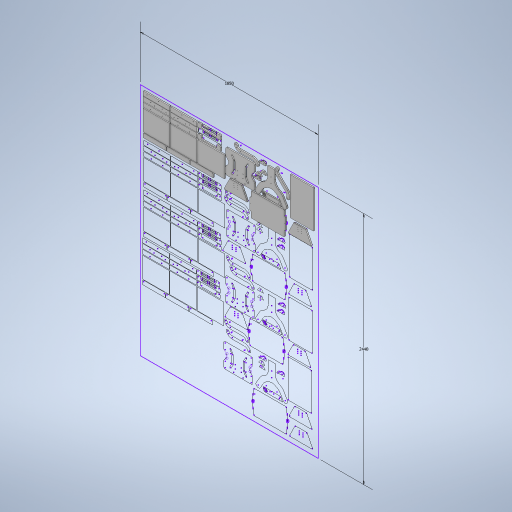
# Autodesk Inventor part: Generador_de_Piezas
Saved by Autodesk Inventor 2024 (Build 280153000, 153)
## iProperties
Created: 2023-05-11
Part Number: Generador_de_Piezas
Material: Genérico
Document SubType Name: Modeling
Designer: sebas
Density: 1 g/cm^3
Appearance: Valor por defecto
Autodesk Inventor part; units mm, degrees
(part 1 of 3)
ref_plane "YZ Plane" through (0, 0, 0) normal (1, 0, 0) x (0, 1, 0)
ref_plane "XZ Plane" through (0, 0, 0) normal (0, 1, 0) x (-1, 0, 0)
ref_plane "XY Plane" through (0, 0, 0) normal (0, 0, 1) x (1, 0, 0)
sketch "Visible" plane through (0, 0, 0) normal (0, 0, 1) x (1, 0, 0)
  line L0 (806.8508, 2400.0345) -> (806.8508, 2412.0345)
  line L1 (646.8508, 2412.0345) -> (619.3508, 2412.0345)
  arc A0 (619.3508, 2412.0345) -> (607.3508, 2400.0345) centre (619.3508, 2400.0345) ccw
  line L2 (646.8508, 2400.0345) -> (646.8508, 2412.0345)
  line L3 (318.2665, 2316.0113) -> (318.2665, 2349.0113)
  line L4 (43.2665, 2316.0113) -> (318.2665, 2316.0113)
  line L5 (43.2665, 2316.0113) -> (43.2665, 2349.0113)
  circle A1 centre (280.5665, 2332.5113) radius 3
  circle A2 centre (160.9665, 2332.5113) radius 3
  circle A3 centre (240.5665, 2343.5113) radius 3
  circle A4 centre (120.9665, 2343.5113) radius 3
  line L6 (318.2665, 2361.0113) -> (318.2665, 2349.0113)
  line L7 (43.2665, 2361.0113) -> (43.2665, 2349.0113)
  line L8 (43.2665, 2361.0113) -> (318.2665, 2361.0113)
  line L9 (600.4289, 2410.0964) -> (600.4289, 2398.0964)
  line L10 (325.4289, 2410.0964) -> (325.4289, 2398.0964)
  line L11 (325.4289, 2410.0964) -> (600.4289, 2410.0964)
  line L12 (600.4289, 2365.0964) -> (600.4289, 2398.0964)
  line L13 (325.4289, 2365.0964) -> (600.4289, 2365.0964)
  line L14 (325.4289, 2365.0964) -> (325.4289, 2398.0964)
  circle A5 centre (562.7289, 2392.5964) radius 3
  circle A6 centre (443.1289, 2392.5964) radius 3
  line L15 (325.2528, 2315.2709) -> (325.2528, 2348.2709)
  line L16 (600.2528, 2315.2709) -> (600.2528, 2348.2709)
  line L17 (600.2528, 2315.2709) -> (325.2528, 2315.2709)
  circle A7 centre (522.5528, 2342.7709) radius 3
  circle A8 centre (402.9528, 2342.7709) radius 3
  circle A9 centre (482.5528, 2331.7709) radius 3
  circle A10 centre (362.9528, 2331.7709) radius 3
  line L18 (325.2528, 2348.2709) -> (325.2528, 2360.2709)
  line L19 (600.2528, 2360.2709) -> (325.2528, 2360.2709)
  line L20 (600.2528, 2348.2709) -> (600.2528, 2360.2709)
  line L21 (799.3625, 2328.4857) -> (659.3625, 2328.4857)
  arc A11 (799.3625, 2328.4857) -> (809.3625, 2338.4857) centre (799.3625, 2338.4857) ccw
  line L22 (809.3625, 2338.4857) -> (809.3625, 2349.4857)
  line L23 (848.8625, 2349.4857) -> (848.8625, 2316.4857)
  line L24 (848.8625, 2316.4857) -> (609.8625, 2316.4857)
  line L25 (609.8625, 2349.4857) -> (609.8625, 2316.4857)
  arc A12 (649.3625, 2338.4857) -> (659.3625, 2328.4857) centre (659.3625, 2338.4857) ccw
  line L26 (649.3625, 2338.4857) -> (649.3625, 2349.4857)
  line L27 (836.8625, 2361.4857) -> (809.3625, 2361.4857)
  arc A13 (848.8625, 2349.4857) -> (836.8625, 2361.4857) centre (836.8625, 2349.4857) ccw
  line L28 (809.3625, 2349.4857) -> (809.3625, 2361.4857)
  line L29 (649.3625, 2361.4857) -> (621.8625, 2361.4857)
  arc A14 (621.8625, 2361.4857) -> (609.8625, 2349.4857) centre (621.8625, 2349.4857) ccw
  line L30 (649.3625, 2349.4857) -> (649.3625, 2361.4857)
  line L31 (42.474, 2263.6267) -> (42.474, 2296.6267)
  line L32 (317.474, 2263.6267) -> (317.474, 2296.6267)
  line L33 (317.474, 2263.6267) -> (42.474, 2263.6267)
  circle A15 centre (239.774, 2280.1267) radius 3
  circle A16 centre (120.174, 2280.1267) radius 3
  line L34 (42.474, 2296.6267) -> (42.474, 2308.6267)
  line L35 (317.474, 2308.6267) -> (42.474, 2308.6267)
  line L36 (317.474, 2296.6267) -> (317.474, 2308.6267)
  line L37 (600.3648, 2308.6267) -> (600.3648, 2296.6267)
  line L38 (325.3648, 2308.6267) -> (325.3648, 2296.6267)
  line L39 (325.3648, 2308.6267) -> (600.3648, 2308.6267)
  line L40 (600.3648, 2263.6267) -> (600.3648, 2296.6267)
  line L41 (325.3648, 2263.6267) -> (600.3648, 2263.6267)
  line L42 (325.3648, 2263.6267) -> (325.3648, 2296.6267)
  circle A17 centre (522.6648, 2280.1267) radius 3
  circle A18 centre (403.0648, 2280.1267) radius 3
  line L43 (797.9907, 2277.247) -> (657.9907, 2277.247)
  arc A19 (797.9907, 2277.247) -> (807.9907, 2287.247) centre (797.9907, 2287.247) ccw
  line L44 (807.9907, 2287.247) -> (807.9907, 2298.247)
  line L45 (847.4907, 2298.247) -> (847.4907, 2265.247)
  line L46 (847.4907, 2265.247) -> (608.4907, 2265.247)
  line L47 (608.4907, 2298.247) -> (608.4907, 2265.247)
  arc A20 (647.9907, 2287.247) -> (657.9907, 2277.247) centre (657.9907, 2287.247) ccw
  line L48 (647.9907, 2287.247) -> (647.9907, 2298.247)
  line L49 (835.4907, 2310.247) -> (807.9907, 2310.247)
  arc A21 (847.4907, 2298.247) -> (835.4907, 2310.247) centre (835.4907, 2298.247) ccw
  line L50 (807.9907, 2298.247) -> (807.9907, 2310.247)
  line L51 (647.9907, 2310.247) -> (620.4907, 2310.247)
  arc A22 (620.4907, 2310.247) -> (608.4907, 2298.247) centre (620.4907, 2298.247) ccw
  line L52 (647.9907, 2298.247) -> (647.9907, 2310.247)
  line L53 (318.3532, 2039.3982) -> (43.3532, 2039.3982)
  line L54 (318.3532, 2039.3982) -> (318.3532, 2254.3982)
  line L55 (43.3532, 2254.3982) -> (43.3532, 2039.3982)
  line L56 (318.3532, 2254.3982) -> (43.3532, 2254.3982)
  line L57 (600.1736, 2040.7797) -> (325.1736, 2040.7797)
  line L58 (600.1736, 2040.7797) -> (600.1736, 2255.7797)
  line L59 (325.1736, 2255.7797) -> (325.1736, 2040.7797)
  line L60 (600.1736, 2255.7797) -> (325.1736, 2255.7797)
  line L61 (885.3014, 2039.5398) -> (610.3014, 2039.5398)
  line L62 (885.3014, 2039.5398) -> (885.3014, 2254.5398)
  line L63 (610.3014, 2254.5398) -> (610.3014, 2039.5398)
  line L64 (885.3014, 2254.5398) -> (610.3014, 2254.5398)
  line L65 (41.6152, 1989.403) -> (280.6152, 1989.403)
  line L66 (41.6152, 2022.403) -> (41.6152, 1989.403)
  line L67 (280.6152, 2022.403) -> (280.6152, 1989.403)
  line L68 (53.6152, 2034.403) -> (268.6152, 2034.403)
  arc A23 (280.6152, 2022.403) -> (268.6152, 2034.403) centre (268.6152, 2022.403) ccw
  arc A24 (53.6152, 2034.403) -> (41.6152, 2022.403) centre (53.6152, 2022.403) ccw
  line L69 (286.1359, 1989.403) -> (525.1359, 1989.403)
  line L70 (286.1359, 2022.403) -> (286.1359, 1989.403)
  line L71 (525.1359, 2022.403) -> (525.1359, 1989.403)
  line L72 (298.1359, 2034.403) -> (513.1359, 2034.403)
  arc A25 (525.1359, 2022.403) -> (513.1359, 2034.403) centre (513.1359, 2022.403) ccw
  arc A26 (298.1359, 2034.403) -> (286.1359, 2022.403) centre (298.1359, 2022.403) ccw
  line L73 (529.3629, 1989.8327) -> (768.3629, 1989.8327)
  line L74 (529.3629, 2022.8327) -> (529.3629, 1989.8327)
  line L75 (768.3629, 2022.8327) -> (768.3629, 1989.8327)
  line L76 (541.3629, 2034.8327) -> (756.3629, 2034.8327)
  arc A27 (768.3629, 2022.8327) -> (756.3629, 2034.8327) centre (756.3629, 2022.8327) ccw
  arc A28 (541.3629, 2034.8327) -> (529.3629, 2022.8327) centre (541.3629, 2022.8327) ccw
  circle A29 centre (717.6352, 2406.9048) radius 3
  circle A30 centre (657.8352, 2406.9048) radius 3
  arc A31 (717.6352, 2401.9048) -> (717.6352, 2411.9048) centre (717.6352, 2406.9048) ccw
  line L77 (717.6352, 2401.9048) -> (657.8352, 2401.9048)
  arc A32 (657.8352, 2411.9048) -> (657.8352, 2401.9048) centre (657.8352, 2406.9048) ccw
  line L78 (717.6352, 2411.9048) -> (657.8352, 2411.9048)
  circle A33 centre (792.7319, 2407.0384) radius 3
  circle A34 centre (732.9319, 2407.0384) radius 3
  arc A35 (792.7319, 2402.0384) -> (792.7319, 2412.0384) centre (792.7319, 2407.0384) ccw
  line L79 (792.7319, 2402.0384) -> (732.9319, 2402.0384)
  arc A36 (732.9319, 2412.0384) -> (732.9319, 2402.0384) centre (732.9319, 2407.0384) ccw
  line L80 (792.7319, 2412.0384) -> (732.9319, 2412.0384)
  circle A37 centre (717.9632, 2391.8594) radius 3
  circle A38 centre (658.1632, 2391.8594) radius 3
  arc A39 (717.9632, 2386.8594) -> (717.9632, 2396.8594) centre (717.9632, 2391.8594) ccw
  line L81 (717.9632, 2386.8594) -> (658.1632, 2386.8594)
  arc A40 (658.1632, 2396.8594) -> (658.1632, 2386.8594) centre (658.1632, 2391.8594) ccw
  line L82 (717.9632, 2396.8594) -> (658.1632, 2396.8594)
  circle A41 centre (793.0598, 2391.993) radius 3
  circle A42 centre (733.2598, 2391.993) radius 3
  arc A43 (793.0598, 2386.993) -> (793.0598, 2396.993) centre (793.0598, 2391.993) ccw
  line L83 (793.0598, 2386.993) -> (733.2598, 2386.993)
  arc A44 (733.2598, 2396.993) -> (733.2598, 2386.993) centre (733.2598, 2391.993) ccw
  line L84 (793.0598, 2396.993) -> (733.2598, 2396.993)
  circle A45 centre (720.4706, 2355.6151) radius 3
  circle A46 centre (660.6706, 2355.6151) radius 3
  arc A47 (720.4706, 2350.6151) -> (720.4706, 2360.6151) centre (720.4706, 2355.6151) ccw
  line L85 (720.4706, 2350.6151) -> (660.6706, 2350.6151)
  arc A48 (660.6706, 2360.6151) -> (660.6706, 2350.6151) centre (660.6706, 2355.6151) ccw
  line L86 (720.4706, 2360.6151) -> (660.6706, 2360.6151)
  circle A49 centre (795.5673, 2355.7486) radius 3
  circle A50 centre (735.7673, 2355.7486) radius 3
  arc A51 (795.5673, 2350.7486) -> (795.5673, 2360.7486) centre (795.5673, 2355.7486) ccw
  line L87 (795.5673, 2350.7486) -> (735.7673, 2350.7486)
  arc A52 (735.7673, 2360.7486) -> (735.7673, 2350.7486) centre (735.7673, 2355.7486) ccw
  line L88 (795.5673, 2360.7486) -> (735.7673, 2360.7486)
  circle A53 centre (720.7986, 2340.5697) radius 3
  circle A54 centre (660.9986, 2340.5697) radius 3
  arc A55 (720.7986, 2335.5697) -> (720.7986, 2345.5697) centre (720.7986, 2340.5697) ccw
  line L89 (720.7986, 2335.5697) -> (660.9986, 2335.5697)
  arc A56 (660.9986, 2345.5697) -> (660.9986, 2335.5697) centre (660.9986, 2340.5697) ccw
  line L90 (720.7986, 2345.5697) -> (660.9986, 2345.5697)
  circle A57 centre (795.8952, 2340.7033) radius 3
  circle A58 centre (736.0952, 2340.7033) radius 3
  arc A59 (795.8952, 2335.7033) -> (795.8952, 2345.7033) centre (795.8952, 2340.7033) ccw
  line L91 (795.8952, 2335.7033) -> (736.0952, 2335.7033)
  arc A60 (736.0952, 2345.7033) -> (736.0952, 2335.7033) centre (736.0952, 2340.7033) ccw
  line L92 (795.8952, 2345.7033) -> (736.0952, 2345.7033)
  circle A61 centre (1238.5575, 2262.083) radius 2.5
  line L93 (1251.0575, 2275.083) -> (1226.0575, 2275.083)
  line L94 (1270.5575, 2247.083) -> (1251.0575, 2275.083)
  line L95 (1206.5575, 2247.083) -> (1270.5575, 2247.083)
  line L96 (1226.0575, 2275.083) -> (1206.5575, 2247.083)
  circle A62 centre (1288.1866, 2298.632) radius 2.5
  line L97 (1300.6866, 2311.632) -> (1275.6866, 2311.632)
  line L98 (1320.1866, 2283.632) -> (1300.6866, 2311.632)
  line L99 (1256.1866, 2283.632) -> (1320.1866, 2283.632)
  line L100 (1275.6866, 2311.632) -> (1256.1866, 2283.632)
  line L101 (1478.5889, 2086.2932) -> (1289.2629, 2086.2932)
  line L102 (1289.2629, 2086.2932) -> (1276.499, 2111.8211)
  arc A63 (1285.4432, 2126.2932) -> (1276.499, 2111.8211) centre (1285.4432, 2116.2932) ccw
  line L103 (1285.4432, 2126.2932) -> (1452.4086, 2126.2932)
  arc A64 (1461.3528, 2120.7653) -> (1452.4086, 2126.2932) centre (1452.4086, 2116.2932) ccw
  line L104 (1478.5889, 2086.2932) -> (1461.3528, 2120.7653)
  circle A65 centre (1446.5889, 2101.2932) radius 2.5
  arc A66 (1291.5413, 2115.3503) -> (1290.9657, 2114.6956) centre (1291.4666, 2114.8356) ccw
  line L105 (1295.6396, 2114.7556) -> (1291.5413, 2115.3503)
  arc A67 (1296.9285, 2111.2385) -> (1295.6396, 2114.7556) centre (1295.3339, 2112.6488) ccw
  arc A68 (1296.9285, 2111.2385) -> (1291.3041, 2103.0866) centre (1300.8635, 2102.5073) ccw
  arc A69 (1291.3041, 2103.0866) -> (1296.9285, 2095.0314) centre (1299.9745, 2103.1494) ccw
  arc A70 (1296.9285, 2095.0314) -> (1305.8519, 2093.2169) centre (1306.0702, 2117.1391) ccw
  arc A71 (1305.8519, 2093.2169) -> (1306.8742, 2098.0799) centre (1306.0926, 2095.7053) ccw
  line L106 (1306.8742, 2098.0799) -> (1297.7224, 2101.0922)
  arc A72 (1299.3863, 2106.4666) -> (1297.7224, 2101.0922) centre (1300.5149, 2103.1724) ccw
  line L107 (1299.3863, 2106.4666) -> (1303.2046, 2105.3242)
  arc A73 (1303.2046, 2105.3242) -> (1304.9194, 2110.2861) centre (1303.9576, 2107.8412) ccw
  line L108 (1304.9194, 2110.2861) -> (1303.368, 2110.8964)
  arc A74 (1303.2046, 2113.5788) -> (1303.368, 2110.8964) centre (1303.9105, 2112.2756) ccw
  line L109 (1303.2046, 2113.5788) -> (1308.0077, 2112.5506)
  arc A75 (1311.3735, 2109.1864) -> (1308.0077, 2112.5506) centre (1307.0908, 2108.2675) ccw
  line L110 (1311.3735, 2109.1864) -> (1313.3885, 2099.7953)
  arc A76 (1313.3885, 2099.7953) -> (1318.892, 2096.3946) centre (1317.7721, 2100.7359) ccw
  arc A77 (1318.892, 2096.3946) -> (1318.892, 2102.1918) centre (1318.1443, 2099.2932) ccw
  line L111 (1318.892, 2102.1918) -> (1317.4612, 2108.8603)
  arc A78 (1317.4612, 2108.8603) -> (1306.7616, 2118.8636) centre (1304.9194, 2106.1693) ccw
  line L112 (1306.7616, 2118.8636) -> (1290.0195, 2121.2932)
  arc A79 (1290.0195, 2121.2932) -> (1288.5063, 2110.8656) centre (1289.2629, 2116.0794) ccw
  arc A80 (1288.5063, 2110.8656) -> (1290.9657, 2114.6956) centre (1288.8653, 2113.3397) ccw
  circle A81 centre (1052.5181, 2370.22) radius 2.5
  circle A82 centre (1226.8114, 2335.22) radius 2.5
  circle A83 centre (1012.5181, 2385.0838) radius 2.5
  arc A84 (1240.9135, 2340.3319) -> (1176.8956, 2385.22) centre (1176.8956, 2317.1259) ccw
  arc A85 (1211.9866, 2332.6383) -> (1240.9135, 2340.3319) centre (1226.7083, 2335.514) ccw
  arc A86 (1211.9866, 2332.6383) -> (1182.3115, 2355.22) centre (1182.3115, 2324.4308) ccw
  line L113 (1048.6669, 2355.22) -> (1182.3115, 2355.22)
  arc A87 (1017.3509, 2407.1763) -> (1042.3844, 2385.22) centre (1042.3844, 2410.4692) ccw
  line L114 (1042.3844, 2385.22) -> (1176.8956, 2385.22)
  circle A88 centre (1002.4791, 2405.22) radius 2.5
  arc A89 (1017.3509, 2407.1763) -> (988.0381, 2401.163) centre (1002.4791, 2405.22) ccw
  arc A90 (988.0381, 2401.163) -> (1048.6669, 2355.22) centre (1048.6669, 2418.196) ccw
  arc A91 (1119.3765, 2256.3016) -> (1118.0367, 2251.3016) centre (1128.0367, 2251.3016) ccw
  arc A92 (1103.3765, 2256.3016) -> (1102.0367, 2251.3016) centre (1112.0367, 2251.3016) ccw
  arc A93 (1102.0367, 2166.6606) -> (1103.3765, 2161.6606) centre (1112.0367, 2166.6606) ccw
  arc A94 (1118.0367, 2166.6606) -> (1119.3765, 2161.6606) centre (1128.0367, 2166.6606) ccw
  arc A95 (1184.5367, 2083.9811) -> (1199.5367, 2098.9811) centre (1184.5367, 2098.9811) ccw
  arc A96 (899.5367, 2098.9811) -> (914.5367, 2083.9811) centre (914.5367, 2098.9811) ccw
  arc A97 (904.9654, 2168.2557) -> (899.5367, 2156.7062) centre (914.5367, 2156.7062) ccw
  arc A98 (899.5367, 2261.256) -> (904.9654, 2249.7066) centre (914.5367, 2261.256) ccw
  arc A99 (914.5367, 2333.9811) -> (899.5367, 2318.9811) centre (914.5367, 2318.9811) ccw
  arc A100 (1199.5367, 2318.9811) -> (1184.5367, 2333.9811) centre (1184.5367, 2318.9811) ccw
  arc A101 (1194.108, 2249.7066) -> (1199.5367, 2261.256) centre (1184.5367, 2261.256) ccw
  arc A102 (1199.5367, 2156.7062) -> (1194.108, 2168.2557) centre (1184.5367, 2156.7062) ccw
  arc A103 (995.697, 2161.6606) -> (997.0367, 2166.6606) centre (987.0367, 2166.6606) ccw
  arc A104 (997.0367, 2251.3016) -> (995.697, 2256.3016) centre (987.0367, 2251.3016) ccw
  arc A105 (981.0367, 2251.3016) -> (979.697, 2256.3016) centre (971.0367, 2251.3016) ccw
  arc A106 (979.697, 2161.6606) -> (981.0367, 2166.6606) centre (971.0367, 2166.6606) ccw
  line L115 (1103.3765, 2161.6606) -> (1125.8207, 2122.786)
  line L116 (979.697, 2161.6606) -> (961.2527, 2129.7143)
  line L117 (1199.5367, 2318.9811) -> (1199.5367, 2261.256)
  circle A107 centre (1019.5367, 2178.9811) radius 2.5
  circle A108 centre (1019.5367, 2138.9811) radius 2.5
  circle A109 centre (999.5367, 2098.9811) radius 4
  circle A110 centre (1099.5367, 2098.9811) radius 4
  circle A111 centre (1079.5367, 2138.9811) radius 2.5
  circle A112 centre (1079.5367, 2178.9811) radius 2.5
  arc A113 (961.2527, 2129.7143) -> (973.2527, 2122.786) centre (967.2527, 2126.2501) ccw
  line L118 (995.697, 2161.6606) -> (973.2527, 2122.786)
  line L119 (997.0367, 2251.3016) -> (997.0367, 2166.6606)
  line L120 (995.697, 2256.3016) -> (973.2527, 2295.1762)
  arc A114 (973.2527, 2295.1762) -> (961.2527, 2288.248) centre (967.2527, 2291.7121) ccw
  line L121 (979.697, 2256.3016) -> (961.2527, 2288.248)
  line L122 (981.0367, 2251.3016) -> (981.0367, 2166.6606)
  spline S0 degree 2 poles (1169.5367, 2208.9811) (1169.5367, 2229.3438) (1194.108, 2249.7066) knots 0.5 0.5 0.5 0.952505 0.952505 0.952505
  line L123 (1169.5367, 2208.9811) -> (1169.5367, 2229.3438) construction
  line L124 (1169.5367, 2229.3438) -> (1194.108, 2249.7066) construction
  spline S1 degree 2 poles (1194.108, 2168.2557) (1169.5367, 2188.6184) (1169.5367, 2208.9811) knots 0.047495 0.047495 0.047495 0.5 0.5 0.5
  line L125 (1194.108, 2168.2557) -> (1169.5367, 2188.6184) construction
  line L126 (1169.5367, 2188.6184) -> (1169.5367, 2208.9811) construction
  line L127 (1199.5367, 2156.7062) -> (1199.5367, 2098.9811)
  line L128 (914.5367, 2083.9811) -> (1184.5367, 2083.9811)
  line L129 (899.5367, 2156.7062) -> (899.5367, 2098.9811)
  spline S2 degree 2 poles (904.9654, 2168.2557) (929.5367, 2188.6184) (929.5367, 2208.9811) knots 0.047495 0.047495 0.047495 0.5 0.5 0.5
  line L130 (904.9654, 2168.2557) -> (929.5367, 2188.6184) construction
  line L131 (929.5367, 2188.6184) -> (929.5367, 2208.9811) construction
  spline S3 degree 2 poles (929.5367, 2208.9811) (929.5367, 2229.3438) (904.9654, 2249.7066) knots 0.5 0.5 0.5 0.952505 0.952505 0.952505
  line L132 (929.5367, 2208.9811) -> (929.5367, 2229.3438) construction
  line L133 (929.5367, 2229.3438) -> (904.9654, 2249.7066) construction
  line L134 (899.5367, 2318.9811) -> (899.5367, 2261.256)
  line L135 (914.5367, 2333.9811) -> (1184.5367, 2333.9811)
  arc A115 (1125.8207, 2122.786) -> (1137.8207, 2129.7143) centre (1131.8207, 2126.2501) ccw
  line L136 (1119.3765, 2161.6606) -> (1137.8207, 2129.7143)
  line L137 (1118.0367, 2251.3016) -> (1118.0367, 2166.6606)
  line L138 (1119.3765, 2256.3016) -> (1137.8207, 2288.248)
  arc A116 (1137.8207, 2288.248) -> (1125.8207, 2295.1762) centre (1131.8207, 2291.7121) ccw
  line L139 (1103.3765, 2256.3016) -> (1125.8207, 2295.1762)
  line L140 (1102.0367, 2251.3016) -> (1102.0367, 2166.6606)
  arc A117 (1489.3759, 2091.2231) -> (1532.6771, 2116.2231) centre (1511.0265, 2103.7231) ccw
  arc A118 (1459.2926, 2143.3289) -> (1430.0105, 2172.611) centre (1390.0105, 2103.3289) ccw
  arc A119 (1411.2348, 2183.4511) -> (1331.2348, 2183.4511) centre (1371.2348, 2114.1691) ccw
  arc A120 (1312.4592, 2172.611) -> (1283.1771, 2143.3289) centre (1352.4592, 2103.3289) ccw
  arc A121 (1209.7926, 2116.2231) -> (1253.0938, 2091.2231) centre (1231.4432, 2103.7231) ccw
  arc A122 (1275.8566, 2209.2135) -> (1246.5746, 2179.9315) centre (1315.8566, 2139.9315) ccw
  arc A123 (1295.2348, 2220.4015) -> (1335.2348, 2289.6835) centre (1255.2348, 2289.6835) ccw
  arc A124 (1407.2348, 2289.6835) -> (1447.2348, 2220.4015) centre (1487.2348, 2289.6835) ccw
  arc A125 (1495.8951, 2179.9315) -> (1466.6131, 2209.2135) centre (1426.6131, 2139.9315) ccw
  circle A126 centre (1371.2348, 2299.1691) radius 2.5
  circle A127 centre (1371.2348, 2239.1691) radius 2.5
  line L141 (1246.5746, 2179.9315) -> (1209.7926, 2116.2231)
  line L142 (1295.2348, 2220.4015) -> (1275.8566, 2209.2135)
  line L143 (1335.2348, 2383.4955) -> (1335.2348, 2289.6835)
  line L144 (1335.2348, 2383.4955) -> (1407.2348, 2383.4955)
  line L145 (1407.2348, 2383.4955) -> (1407.2348, 2289.6835)
  line L146 (1447.2348, 2220.4015) -> (1466.6131, 2209.2135)
  line L147 (1495.8951, 2179.9315) -> (1532.6771, 2116.2231)
  line L148 (1489.3759, 2091.2231) -> (1459.2926, 2143.3289)
  line L149 (1430.0105, 2172.611) -> (1411.2348, 2183.4511)
  line L150 (1312.4592, 2172.611) -> (1331.2348, 2183.4511)
  line L151 (1253.0938, 2091.2231) -> (1283.1771, 2143.3289)
  arc A128 (1199.8313, 2215.0969) -> (1209.4145, 2222.2398) centre (1199.8313, 2225.0969) ccw
  arc A129 (1210.5802, 2225.3692) -> (1209.4145, 2222.2398) centre (1233.3723, 2215.0969) ccw
  line L152 (1212.6368, 2224.1819) -> (1210.5802, 2225.3692)
  arc A130 (1212.6368, 2224.1819) -> (1215.1368, 2228.512) centre (1213.8868, 2226.3469) ccw
  line L153 (1215.1368, 2228.512) -> (1213.0802, 2229.6993)
  arc A131 (1218.7699, 2235.389) -> (1213.0802, 2229.6993) centre (1233.3723, 2215.0969) ccw
  line L154 (1219.9573, 2233.3325) -> (1218.7699, 2235.389)
  arc A132 (1219.9573, 2233.3325) -> (1224.2874, 2235.8325) centre (1222.1223, 2234.5825) ccw
  line L155 (1224.2874, 2235.8325) -> (1223.1001, 2237.889)
  arc A133 (1230.8723, 2239.9716) -> (1223.1001, 2237.889) centre (1233.3723, 2215.0969) ccw
  line L156 (1230.8723, 2237.5969) -> (1230.8723, 2239.9716)
  arc A134 (1230.8723, 2237.5969) -> (1235.8723, 2237.5969) centre (1233.3723, 2237.5969) ccw
  line L157 (1235.8723, 2237.5969) -> (1235.8723, 2239.9716)
  arc A135 (1243.6446, 2237.889) -> (1235.8723, 2239.9716) centre (1233.3723, 2215.0969) ccw
  line L158 (1242.4573, 2235.8325) -> (1243.6446, 2237.889)
  arc A136 (1242.4573, 2235.8325) -> (1246.7874, 2233.3325) centre (1244.6223, 2234.5825) ccw
  line L159 (1246.7874, 2233.3325) -> (1247.9748, 2235.389)
  arc A137 (1253.6645, 2229.6993) -> (1247.9748, 2235.389) centre (1233.3723, 2215.0969) ccw
  line L160 (1251.6079, 2228.512) -> (1253.6645, 2229.6993)
  arc A138 (1251.6079, 2228.512) -> (1254.1079, 2224.1819) centre (1252.8579, 2226.3469) ccw
  line L161 (1254.1079, 2224.1819) -> (1256.1645, 2225.3692)
  arc A139 (1256.2852, 2205.0969) -> (1256.1645, 2225.3692) centre (1233.3723, 2215.0969) ccw
  line L162 (1178.3723, 2205.0969) -> (1256.2852, 2205.0969)
  arc A140 (1188.3723, 2215.0969) -> (1178.3723, 2205.0969) centre (1188.3723, 2205.0969) ccw
  line L163 (1188.3723, 2215.0969) -> (1199.8313, 2215.0969)
  circle A141 centre (1233.3723, 2215.0969) radius 2.5
  line L164 (1062.9808, 2071.3053) -> (945.8278, 2071.3053)
  circle A142 centre (1022.9043, 2046.1862) radius 1.5
  circle A143 centre (1022.9043, 2010.9481) radius 1.5
  circle A144 centre (985.9043, 2010.9481) radius 1.5
  circle A145 centre (985.9043, 2028.5672) radius 1.5
  circle A146 centre (985.9043, 2046.1862) radius 1.5
  circle A147 centre (1022.9043, 2028.5672) radius 1.5
  line L165 (889.1611, 1947.972) -> (1119.6474, 1947.972)
  line L166 (941.3556, 2068.5414) -> (884.689, 1955.208)
  line L167 (1124.1196, 1955.208) -> (1067.4529, 2068.5414)
  arc A148 (884.6942, 1955.2184) -> (889.1667, 1947.972) centre (889.1611, 1952.972) ccw
  arc A149 (1119.6358, 1947.972) -> (1124.1171, 1955.213) centre (1119.6474, 1952.972) ccw
  arc A150 (945.8314, 2071.3053) -> (941.3552, 2068.5404) centre (945.8278, 2066.3053) ccw
  arc A151 (1067.4545, 2068.5381) -> (1062.9797, 2071.3053) centre (1062.9808, 2066.3053) ccw
  line L168 (1157.0805, 2012.1486) -> (1156.654, 2012.1486)
  line L169 (1151.0805, 1894.8152) -> (1151.0805, 2006.1486)
  line L170 (1163.4138, 1833.1486) -> (1163.4138, 1882.8152)
  line L171 (1169.4138, 2073.8152) -> (1502.7472, 2073.8152)
  line L172 (1508.7472, 1882.8152) -> (1508.7472, 1833.1486)
  line L173 (1508.7472, 2067.8152) -> (1508.7472, 2018.1486)
  line L174 (1163.4138, 2018.9084) -> (1163.4138, 2067.8152)
  line L175 (1502.7472, 1827.1486) -> (1169.4138, 1827.1486)
  line L176 (1514.7472, 2012.1486) -> (1515.0805, 2012.1486)
  line L177 (1157.4138, 1888.8152) -> (1157.0805, 1888.8152)
  line L178 (1521.0805, 2006.1486) -> (1521.0805, 1894.8152)
  line L179 (1515.0805, 1888.8152) -> (1514.7472, 1888.8152)
  arc A152 (1157.0805, 2012.1486) -> (1153.2015, 2010.7261) centre (1157.0805, 2006.1486) ccw
  arc A153 (1153.2015, 2010.7261) -> (1156.0806, 2007.1627) centre (1174.1634, 2024.7173) ccw
  spline S4 degree 3 poles (1516.0805, 1943.9819) (1516.0822, 1943.9834) (1516.1095, 1944.008) (1518.4407, 1946.5739) (1519.1702, 1948.7405) (1519.4137, 1950.636) (1519.107, 1952.4883) (1518.1671, 1954.7656) (1516.1084, 1956.9556) (1516.0823, 1956.9802) (1516.0805, 1956.9819) knots 0 0 0 0 0.01236 0.196358 0.365814 0.504316 0.642688 0.817015 0.98764 1 1 1 1
  line L180 (1516.0805, 1943.9819) -> (1516.0822, 1943.9834) construction
  line L181 (1516.0822, 1943.9834) -> (1516.1095, 1944.008) construction
  line L182 (1516.1095, 1944.008) -> (1518.4407, 1946.5739) construction
  line L183 (1518.4407, 1946.5739) -> (1519.1702, 1948.7405) construction
  line L184 (1519.1702, 1948.7405) -> (1519.4137, 1950.636) construction
  line L185 (1519.4137, 1950.636) -> (1519.107, 1952.4883) construction
  line L186 (1519.107, 1952.4883) -> (1518.1671, 1954.7656) construction
  line L187 (1518.1671, 1954.7656) -> (1516.1084, 1956.9556) construction
  line L188 (1516.1084, 1956.9556) -> (1516.0823, 1956.9802) construction
  line L189 (1516.0823, 1956.9802) -> (1516.0805, 1956.9819) construction
  arc A154 (1153.2015, 2010.7261) -> (1151.0805, 2006.1486) centre (1157.0805, 2006.1486) ccw
  spline S5 degree 3 poles (1156.0805, 1943.9819) (1156.0787, 1943.9836) (1156.0525, 1944.0082) (1153.9939, 1946.1982) (1153.054, 1948.4755) (1152.7473, 1950.3278) (1152.9908, 1952.2233) (1153.7202, 1954.3899) (1156.0515, 1956.9558) (1156.0788, 1956.9803) (1156.0805, 1956.9819) knots 0 0 0 0 0.01236 0.182985 0.357312 0.495684 0.634186 0.803642 0.98764 1 1 1 1
  line L190 (1156.0805, 1943.9819) -> (1156.0787, 1943.9836) construction
  line L191 (1156.0787, 1943.9836) -> (1156.0525, 1944.0082) construction
  line L192 (1156.0525, 1944.0082) -> (1153.9939, 1946.1982) construction
  line L193 (1153.9939, 1946.1982) -> (1153.054, 1948.4755) construction
  line L194 (1153.054, 1948.4755) -> (1152.7473, 1950.3278) construction
  line L195 (1152.7473, 1950.3278) -> (1152.9908, 1952.2233) construction
  line L196 (1152.9908, 1952.2233) -> (1153.7202, 1954.3899) construction
  line L197 (1153.7202, 1954.3899) -> (1156.0515, 1956.9558) construction
  line L198 (1156.0515, 1956.9558) -> (1156.0788, 1956.9803) construction
  line L199 (1156.0788, 1956.9803) -> (1156.0805, 1956.9819) construction
  arc A155 (1156.654, 2012.1486) -> (1163.4138, 2018.9084) centre (1156.654, 2018.9084) ccw
  arc A156 (1151.0805, 1894.8152) -> (1157.0805, 1888.8152) centre (1157.0805, 1894.8152) ccw
  circle A157 centre (1156.0805, 1950.4819) radius 1.5
  arc A158 (1163.4138, 1833.1486) -> (1169.4138, 1827.1486) centre (1169.4138, 1833.1486) ccw
  arc A159 (1508.7472, 2018.1486) -> (1514.7472, 2012.1486) centre (1514.7472, 2018.1486) ccw
  arc A160 (1502.7472, 1827.1486) -> (1508.7472, 1833.1486) centre (1502.7472, 1833.1486) ccw
  circle A161 centre (1516.0805, 1950.4819) radius 1.5
  arc A162 (1163.4138, 1882.8152) -> (1157.4138, 1888.8152) centre (1157.4138, 1882.8152) ccw
  arc A163 (1508.7472, 2067.8152) -> (1502.7472, 2073.8152) centre (1502.7472, 2067.8152) ccw
  arc A164 (1169.4138, 2073.8152) -> (1163.4138, 2067.8152) centre (1169.4138, 2067.8152) ccw
  arc A165 (1521.0805, 2006.1486) -> (1515.0805, 2012.1486) centre (1515.0805, 2006.1486) ccw
  arc A166 (1514.7472, 1888.8152) -> (1508.7472, 1882.8152) centre (1514.7472, 1882.8152) ccw
  arc A167 (1515.0805, 1888.8152) -> (1521.0805, 1894.8152) centre (1515.0805, 1894.8152) ccw
  line L200 (1573.6533, 2032.2187) -> (1810.3199, 2032.2187)
  line L201 (1810.3199, 2422.2187) -> (1573.6533, 2422.2187)
  line L202 (1815.3199, 2037.2187) -> (1815.3199, 2417.2187)
  line L203 (1568.6533, 2417.2187) -> (1568.6533, 2037.2187)
  arc A168 (1568.6533, 2037.2227) -> (1573.6541, 2032.2187) centre (1573.6533, 2037.2187) ccw
  arc A169 (1810.316, 2032.2187) -> (1815.3199, 2037.2183) centre (1810.3199, 2037.2187) ccw
  arc A170 (1815.3199, 2417.216) -> (1810.3203, 2422.2187) centre (1810.3199, 2417.2187) ccw
  arc A171 (1573.6572, 2422.2187) -> (1568.6533, 2417.2191) centre (1573.6533, 2417.2187) ccw
  line L204 (1728.414, 2007.8028) -> (1611.261, 2007.8028)
  circle A172 centre (1688.3375, 1982.6837) radius 1.5
  circle A173 centre (1688.3375, 1947.4456) radius 1.5
  circle A174 centre (1651.3375, 1947.4456) radius 1.5
  circle A175 centre (1651.3375, 1965.0647) radius 1.5
  circle A176 centre (1651.3375, 1982.6837) radius 1.5
  circle A177 centre (1688.3375, 1965.0647) radius 1.5
  line L205 (1554.5943, 1884.4694) -> (1785.0807, 1884.4694)
  line L206 (1606.7889, 2005.0388) -> (1550.1222, 1891.7055)
  line L207 (1789.5528, 1891.7055) -> (1732.8861, 2005.0388)
  arc A178 (1550.1274, 1891.7159) -> (1554.5999, 1884.4694) centre (1554.5943, 1889.4694) ccw
  arc A179 (1785.069, 1884.4694) -> (1789.5503, 1891.7105) centre (1785.0807, 1889.4694) ccw
  arc A180 (1611.2646, 2007.8028) -> (1606.7884, 2005.0379) centre (1611.261, 2002.8028) ccw
  arc A181 (1732.8877, 2005.0356) -> (1728.413, 2007.8028) centre (1728.414, 2002.8028) ccw
  circle A182 centre (1240.1593, 1755.5273) radius 2.5
  line L208 (1252.6593, 1768.5273) -> (1227.6593, 1768.5273)
  line L209 (1272.1593, 1740.5273) -> (1252.6593, 1768.5273)
  line L210 (1208.1593, 1740.5273) -> (1272.1593, 1740.5273)
  line L211 (1227.6593, 1768.5273) -> (1208.1593, 1740.5273)
  circle A183 centre (1237.4858, 1798.825) radius 2.5
  line L212 (1249.9858, 1811.825) -> (1224.9858, 1811.825)
  line L213 (1269.4858, 1783.825) -> (1249.9858, 1811.825)
  line L214 (1205.4858, 1783.825) -> (1269.4858, 1783.825)
  line L215 (1224.9858, 1811.825) -> (1205.4858, 1783.825)
  line L216 (1460.6469, 1508.6752) -> (1271.3209, 1508.6752)
  line L217 (1271.3209, 1508.6752) -> (1258.5569, 1534.2031)
  arc A184 (1267.5012, 1548.6752) -> (1258.5569, 1534.2031) centre (1267.5012, 1538.6752) ccw
  line L218 (1267.5012, 1548.6752) -> (1434.4665, 1548.6752)
  arc A185 (1443.4108, 1543.1474) -> (1434.4665, 1548.6752) centre (1434.4665, 1538.6752) ccw
  line L219 (1460.6469, 1508.6752) -> (1443.4108, 1543.1474)
  circle A186 centre (1428.6469, 1523.6752) radius 2.5
  arc A187 (1273.5992, 1537.7323) -> (1273.0236, 1537.0776) centre (1273.5245, 1537.2176) ccw
  line L220 (1277.6976, 1537.1376) -> (1273.5992, 1537.7323)
  arc A188 (1278.9864, 1533.6205) -> (1277.6976, 1537.1376) centre (1277.3918, 1535.0309) ccw
  arc A189 (1278.9864, 1533.6205) -> (1273.3621, 1525.4687) centre (1282.9214, 1524.8894) ccw
  arc A190 (1273.3621, 1525.4687) -> (1278.9864, 1517.4135) centre (1282.0324, 1525.5314) ccw
  arc A191 (1278.9864, 1517.4135) -> (1287.9098, 1515.5989) centre (1288.1282, 1539.5211) ccw
  arc A192 (1287.9098, 1515.5989) -> (1288.9322, 1520.462) centre (1288.1505, 1518.0873) ccw
  line L221 (1288.9322, 1520.462) -> (1279.7803, 1523.4742)
  arc A193 (1281.4443, 1528.8486) -> (1279.7803, 1523.4742) centre (1282.5728, 1525.5544) ccw
  line L222 (1281.4443, 1528.8486) -> (1285.2625, 1527.7062)
  arc A194 (1285.2625, 1527.7062) -> (1286.9774, 1532.6682) centre (1286.0156, 1530.2233) ccw
  line L223 (1286.9774, 1532.6682) -> (1285.4259, 1533.2784)
  arc A195 (1285.2625, 1535.9608) -> (1285.4259, 1533.2784) centre (1285.9685, 1534.6577) ccw
  line L224 (1285.2625, 1535.9608) -> (1290.0656, 1534.9327)
  arc A196 (1293.4315, 1531.5685) -> (1290.0656, 1534.9327) centre (1289.1488, 1530.6495) ccw
  line L225 (1293.4315, 1531.5685) -> (1295.4465, 1522.1773)
  arc A197 (1295.4465, 1522.1773) -> (1300.95, 1518.7766) centre (1299.8301, 1523.1179) ccw
  arc A198 (1300.95, 1518.7766) -> (1300.95, 1524.5738) centre (1300.2022, 1521.6752) ccw
  line L226 (1300.95, 1524.5738) -> (1299.5191, 1531.2424)
  arc A199 (1299.5191, 1531.2424) -> (1288.8196, 1541.2456) centre (1286.9774, 1528.5513) ccw
  line L227 (1288.8196, 1541.2456) -> (1272.0775, 1543.6752)
  arc A200 (1272.0775, 1543.6752) -> (1270.5642, 1533.2476) centre (1271.3209, 1538.4614) ccw
  arc A201 (1270.5642, 1533.2476) -> (1273.0236, 1537.0776) centre (1270.9233, 1535.7217) ccw
  circle A202 centre (945.6731, 1884.852) radius 2.5
  circle A203 centre (1119.9664, 1849.852) radius 2.5
  circle A204 centre (905.6731, 1899.7158) radius 2.5
  arc A205 (1134.0684, 1854.9639) -> (1070.0506, 1899.852) centre (1070.0506, 1831.7579) ccw
  arc A206 (1105.1415, 1847.2703) -> (1134.0684, 1854.9639) centre (1119.8633, 1850.146) ccw
  arc A207 (1105.1415, 1847.2703) -> (1075.4664, 1869.852) centre (1075.4664, 1839.0628) ccw
  line L228 (941.8219, 1869.852) -> (1075.4664, 1869.852)
  arc A208 (910.5059, 1921.8083) -> (935.5394, 1899.852) centre (935.5394, 1925.1012) ccw
  line L229 (935.5394, 1899.852) -> (1070.0506, 1899.852)
  circle A209 centre (895.634, 1919.852) radius 2.5
  arc A210 (910.5059, 1921.8083) -> (881.1931, 1915.795) centre (895.634, 1919.852) ccw
  arc A211 (881.1931, 1915.795) -> (941.8219, 1869.852) centre (941.8219, 1932.828) ccw
  arc A212 (1115.4652, 1693.168) -> (1114.1255, 1688.168) centre (1124.1255, 1688.168) ccw
  arc A213 (1099.4652, 1693.168) -> (1098.1255, 1688.168) centre (1108.1255, 1688.168) ccw
  arc A214 (1098.1255, 1603.527) -> (1099.4652, 1598.527) centre (1108.1255, 1603.527) ccw
  arc A215 (1114.1255, 1603.527) -> (1115.4652, 1598.527) centre (1124.1255, 1603.527) ccw
  arc A216 (1180.6255, 1520.8475) -> (1195.6255, 1535.8475) centre (1180.6255, 1535.8475) ccw
  arc A217 (895.6255, 1535.8475) -> (910.6255, 1520.8475) centre (910.6255, 1535.8475) ccw
  arc A218 (901.0542, 1605.122) -> (895.6255, 1593.5726) centre (910.6255, 1593.5726) ccw
  arc A219 (895.6255, 1698.1224) -> (901.0542, 1686.5729) centre (910.6255, 1698.1224) ccw
  arc A220 (910.6255, 1770.8475) -> (895.6255, 1755.8475) centre (910.6255, 1755.8475) ccw
  arc A221 (1195.6255, 1755.8475) -> (1180.6255, 1770.8475) centre (1180.6255, 1755.8475) ccw
  arc A222 (1190.1968, 1686.5729) -> (1195.6255, 1698.1224) centre (1180.6255, 1698.1224) ccw
  arc A223 (1195.6255, 1593.5726) -> (1190.1968, 1605.122) centre (1180.6255, 1593.5726) ccw
  arc A224 (991.7857, 1598.527) -> (993.1255, 1603.527) centre (983.1255, 1603.527) ccw
  arc A225 (993.1255, 1688.168) -> (991.7857, 1693.168) centre (983.1255, 1688.168) ccw
  arc A226 (977.1255, 1688.168) -> (975.7857, 1693.168) centre (967.1255, 1688.168) ccw
  arc A227 (975.7857, 1598.527) -> (977.1255, 1603.527) centre (967.1255, 1603.527) ccw
  line L230 (1099.4652, 1598.527) -> (1121.9094, 1559.6524)
  line L231 (975.7857, 1598.527) -> (957.3415, 1566.5806)
  line L232 (1195.6255, 1755.8475) -> (1195.6255, 1698.1224)
  circle A228 centre (1015.6255, 1615.8475) radius 2.5
  circle A229 centre (1015.6255, 1575.8475) radius 2.5
  circle A230 centre (995.6255, 1535.8475) radius 4
  circle A231 centre (1095.6255, 1535.8475) radius 4
  circle A232 centre (1075.6255, 1575.8475) radius 2.5
  circle A233 centre (1075.6255, 1615.8475) radius 2.5
  arc A234 (957.3415, 1566.5806) -> (969.3415, 1559.6524) centre (963.3415, 1563.1165) ccw
  line L233 (991.7857, 1598.527) -> (969.3415, 1559.6524)
  line L234 (993.1255, 1688.168) -> (993.1255, 1603.527)
  line L235 (991.7857, 1693.168) -> (969.3415, 1732.0425)
  arc A235 (969.3415, 1732.0425) -> (957.3415, 1725.1143) centre (963.3415, 1728.5784) ccw
  line L236 (975.7857, 1693.168) -> (957.3415, 1725.1143)
  line L237 (977.1255, 1688.168) -> (977.1255, 1603.527)
  spline S6 degree 2 poles (1165.6255, 1645.8475) (1165.6255, 1666.2102) (1190.1968, 1686.5729) knots 0.5 0.5 0.5 0.952505 0.952505 0.952505
  line L238 (1165.6255, 1645.8475) -> (1165.6255, 1666.2102) construction
  line L239 (1165.6255, 1666.2102) -> (1190.1968, 1686.5729) construction
  spline S7 degree 2 poles (1190.1968, 1605.122) (1165.6255, 1625.4848) (1165.6255, 1645.8475) knots 0.047495 0.047495 0.047495 0.5 0.5 0.5
  line L240 (1190.1968, 1605.122) -> (1165.6255, 1625.4848) construction
  line L241 (1165.6255, 1625.4848) -> (1165.6255, 1645.8475) construction
  line L242 (1195.6255, 1593.5726) -> (1195.6255, 1535.8475)
  line L243 (910.6255, 1520.8475) -> (1180.6255, 1520.8475)
  line L244 (895.6255, 1593.5726) -> (895.6255, 1535.8475)
  spline S8 degree 2 poles (901.0542, 1605.122) (925.6255, 1625.4848) (925.6255, 1645.8475) knots 0.047495 0.047495 0.047495 0.5 0.5 0.5
  line L245 (901.0542, 1605.122) -> (925.6255, 1625.4848) construction
  line L246 (925.6255, 1625.4848) -> (925.6255, 1645.8475) construction
  spline S9 degree 2 poles (925.6255, 1645.8475) (925.6255, 1666.2102) (901.0542, 1686.5729) knots 0.5 0.5 0.5 0.952505 0.952505 0.952505
  line L247 (925.6255, 1645.8475) -> (925.6255, 1666.2102) construction
  line L248 (925.6255, 1666.2102) -> (901.0542, 1686.5729) construction
  line L249 (895.6255, 1755.8475) -> (895.6255, 1698.1224)
  line L250 (910.6255, 1770.8475) -> (1180.6255, 1770.8475)
  arc A236 (1121.9094, 1559.6524) -> (1133.9094, 1566.5806) centre (1127.9094, 1563.1165) ccw
  line L251 (1115.4652, 1598.527) -> (1133.9094, 1566.5806)
  line L252 (1114.1255, 1688.168) -> (1114.1255, 1603.527)
  line L253 (1115.4652, 1693.168) -> (1133.9094, 1725.1143)
  arc A237 (1133.9094, 1725.1143) -> (1121.9094, 1732.0425) centre (1127.9094, 1728.5784) ccw
  line L254 (1099.4652, 1693.168) -> (1121.9094, 1732.0425)
  line L255 (1098.1255, 1688.168) -> (1098.1255, 1603.527)
  arc A238 (1483.344, 1528.7652) -> (1526.6453, 1553.7652) centre (1504.9947, 1541.2652) ccw
  arc A239 (1453.2607, 1580.871) -> (1423.9787, 1610.153) centre (1383.9787, 1540.871) ccw
  arc A240 (1405.203, 1620.9932) -> (1325.203, 1620.9932) centre (1365.203, 1551.7111) ccw
  arc A241 (1306.4273, 1610.153) -> (1277.1453, 1580.871) centre (1346.4273, 1540.871) ccw
  arc A242 (1203.7607, 1553.7652) -> (1247.062, 1528.7652) centre (1225.4114, 1541.2652) ccw
  arc A243 (1269.8248, 1646.7556) -> (1240.5428, 1617.4735) centre (1309.8248, 1577.4735) ccw
  arc A244 (1289.203, 1657.9436) -> (1329.203, 1727.2256) centre (1249.203, 1727.2256) ccw
  arc A245 (1401.203, 1727.2256) -> (1441.203, 1657.9436) centre (1481.203, 1727.2256) ccw
  arc A246 (1489.8633, 1617.4735) -> (1460.5813, 1646.7556) centre (1420.5813, 1577.4735) ccw
  circle A247 centre (1365.203, 1736.7111) radius 2.5
  circle A248 centre (1365.203, 1676.7111) radius 2.5
  line L256 (1240.5428, 1617.4735) -> (1203.7607, 1553.7652)
  line L257 (1289.203, 1657.9436) -> (1269.8248, 1646.7556)
  line L258 (1329.203, 1821.0376) -> (1329.203, 1727.2256)
  line L259 (1329.203, 1821.0376) -> (1401.203, 1821.0376)
  line L260 (1401.203, 1821.0376) -> (1401.203, 1727.2256)
  line L261 (1441.203, 1657.9436) -> (1460.5813, 1646.7556)
  line L262 (1489.8633, 1617.4735) -> (1526.6453, 1553.7652)
  line L263 (1483.344, 1528.7652) -> (1453.2607, 1580.871)
  line L264 (1423.9787, 1610.153) -> (1405.203, 1620.9932)
  line L265 (1306.4273, 1610.153) -> (1325.203, 1620.9932)
  line L266 (1247.062, 1528.7652) -> (1277.1453, 1580.871)
  arc A249 (1446.0743, 1770.9669) -> (1455.6575, 1778.1097) centre (1446.0743, 1780.9669) ccw
  arc A250 (1456.8232, 1781.2391) -> (1455.6575, 1778.1097) centre (1479.6153, 1770.9669) ccw
  line L267 (1458.8798, 1780.0518) -> (1456.8232, 1781.2391)
  arc A251 (1458.8798, 1780.0518) -> (1461.3798, 1784.3819) centre (1460.1298, 1782.2169) ccw
  line L268 (1461.3798, 1784.3819) -> (1459.3232, 1785.5693)
  arc A252 (1465.0129, 1791.259) -> (1459.3232, 1785.5693) centre (1479.6153, 1770.9669) ccw
  line L269 (1466.2003, 1789.2024) -> (1465.0129, 1791.259)
  arc A253 (1466.2003, 1789.2024) -> (1470.5304, 1791.7024) centre (1468.3653, 1790.4524) ccw
  line L270 (1470.5304, 1791.7024) -> (1469.3431, 1793.759)
  arc A254 (1477.1153, 1795.8415) -> (1469.3431, 1793.759) centre (1479.6153, 1770.9669) ccw
  line L271 (1477.1153, 1793.4669) -> (1477.1153, 1795.8415)
  arc A255 (1477.1153, 1793.4669) -> (1482.1153, 1793.4669) centre (1479.6153, 1793.4669) ccw
  line L272 (1482.1153, 1793.4669) -> (1482.1153, 1795.8415)
  arc A256 (1489.8876, 1793.759) -> (1482.1153, 1795.8415) centre (1479.6153, 1770.9669) ccw
  line L273 (1488.7003, 1791.7024) -> (1489.8876, 1793.759)
  arc A257 (1488.7003, 1791.7024) -> (1493.0304, 1789.2024) centre (1490.8653, 1790.4524) ccw
  line L274 (1493.0304, 1789.2024) -> (1494.2178, 1791.259)
  arc A258 (1499.9075, 1785.5693) -> (1494.2178, 1791.259) centre (1479.6153, 1770.9669) ccw
  line L275 (1497.8509, 1784.3819) -> (1499.9075, 1785.5693)
  arc A259 (1497.8509, 1784.3819) -> (1500.3509, 1780.0518) centre (1499.1009, 1782.2169) ccw
  line L276 (1500.3509, 1780.0518) -> (1502.4075, 1781.2391)
  arc A260 (1502.5282, 1760.9669) -> (1502.4075, 1781.2391) centre (1479.6153, 1770.9669) ccw
  line L277 (1424.6153, 1760.9669) -> (1502.5282, 1760.9669)
  arc A261 (1434.6153, 1770.9669) -> (1424.6153, 1760.9669) centre (1434.6153, 1760.9669) ccw
  line L278 (1434.6153, 1770.9669) -> (1446.0743, 1770.9669)
  circle A262 centre (1479.6153, 1770.9669) radius 2.5
  line L279 (1155.8447, 1436.8651) -> (1155.4182, 1436.8651)
  line L280 (1149.8447, 1319.5318) -> (1149.8447, 1430.8651)
  line L281 (1162.178, 1257.8651) -> (1162.178, 1307.5318)
  line L282 (1168.178, 1498.5318) -> (1501.5113, 1498.5318)
  line L283 (1507.5113, 1307.5318) -> (1507.5113, 1257.8651)
  line L284 (1507.5113, 1492.5318) -> (1507.5113, 1442.8651)
  line L285 (1162.178, 1443.6249) -> (1162.178, 1492.5318)
  line L286 (1501.5113, 1251.8651) -> (1168.178, 1251.8651)
  line L287 (1513.5113, 1436.8651) -> (1513.8447, 1436.8651)
  line L288 (1156.178, 1313.5318) -> (1155.8447, 1313.5318)
  line L289 (1519.8447, 1430.8651) -> (1519.8447, 1319.5318)
  line L290 (1513.8447, 1313.5318) -> (1513.5113, 1313.5318)
  arc A263 (1155.8447, 1436.8651) -> (1151.9657, 1435.4426) centre (1155.8447, 1430.8651) ccw
  arc A264 (1151.9657, 1435.4426) -> (1154.8448, 1431.8792) centre (1172.9275, 1449.4338) ccw
  spline S10 degree 3 poles (1514.8447, 1368.6984) (1514.8464, 1368.7) (1514.8736, 1368.7246) (1517.2049, 1371.2904) (1517.9343, 1373.4571) (1518.1779, 1375.3525) (1517.8712, 1377.2048) (1516.9312, 1379.4821) (1514.8726, 1381.6721) (1514.8464, 1381.6968) (1514.8447, 1381.6984) knots 0 0 0 0 0.01236 0.196358 0.365814 0.504316 0.642688 0.817015 0.98764 1 1 1 1
  line L291 (1514.8447, 1368.6984) -> (1514.8464, 1368.7) construction
  line L292 (1514.8464, 1368.7) -> (1514.8736, 1368.7246) construction
  line L293 (1514.8736, 1368.7246) -> (1517.2049, 1371.2904) construction
  line L294 (1517.2049, 1371.2904) -> (1517.9343, 1373.4571) construction
  line L295 (1517.9343, 1373.4571) -> (1518.1779, 1375.3525) construction
  line L296 (1518.1779, 1375.3525) -> (1517.8712, 1377.2048) construction
  line L297 (1517.8712, 1377.2048) -> (1516.9312, 1379.4821) construction
  line L298 (1516.9312, 1379.4821) -> (1514.8726, 1381.6721) construction
  line L299 (1514.8726, 1381.6721) -> (1514.8464, 1381.6968) construction
  line L300 (1514.8464, 1381.6968) -> (1514.8447, 1381.6984) construction
  arc A265 (1151.9657, 1435.4426) -> (1149.8447, 1430.8651) centre (1155.8447, 1430.8651) ccw
  spline S11 degree 3 poles (1154.8447, 1368.6984) (1154.8429, 1368.7001) (1154.8167, 1368.7248) (1152.7581, 1370.9148) (1151.8181, 1373.1921) (1151.5114, 1375.0444) (1151.755, 1376.9398) (1152.4844, 1379.1064) (1154.8157, 1381.6723) (1154.8429, 1381.6969) (1154.8447, 1381.6984) knots 0 0 0 0 0.01236 0.182985 0.357312 0.495684 0.634186 0.803642 0.98764 1 1 1 1
  line L301 (1154.8447, 1368.6984) -> (1154.8429, 1368.7001) construction
  line L302 (1154.8429, 1368.7001) -> (1154.8167, 1368.7248) construction
  line L303 (1154.8167, 1368.7248) -> (1152.7581, 1370.9148) construction
  line L304 (1152.7581, 1370.9148) -> (1151.8181, 1373.1921) construction
  line L305 (1151.8181, 1373.1921) -> (1151.5114, 1375.0444) construction
  line L306 (1151.5114, 1375.0444) -> (1151.755, 1376.9398) construction
  line L307 (1151.755, 1376.9398) -> (1152.4844, 1379.1064) construction
  line L308 (1152.4844, 1379.1064) -> (1154.8157, 1381.6723) construction
  line L309 (1154.8157, 1381.6723) -> (1154.8429, 1381.6969) construction
  line L310 (1154.8429, 1381.6969) -> (1154.8447, 1381.6984) construction
  arc A266 (1155.4182, 1436.8651) -> (1162.178, 1443.6249) centre (1155.4182, 1443.6249) ccw
  arc A267 (1149.8447, 1319.5318) -> (1155.8447, 1313.5318) centre (1155.8447, 1319.5318) ccw
  circle A268 centre (1154.8447, 1375.1984) radius 1.5
  arc A269 (1162.178, 1257.8651) -> (1168.178, 1251.8651) centre (1168.178, 1257.8651) ccw
  arc A270 (1507.5113, 1442.8651) -> (1513.5113, 1436.8651) centre (1513.5113, 1442.8651) ccw
  arc A271 (1501.5113, 1251.8651) -> (1507.5113, 1257.8651) centre (1501.5113, 1257.8651) ccw
  circle A272 centre (1514.8447, 1375.1984) radius 1.5
  arc A273 (1162.178, 1307.5318) -> (1156.178, 1313.5318) centre (1156.178, 1307.5318) ccw
  arc A274 (1507.5113, 1492.5318) -> (1501.5113, 1498.5318) centre (1501.5113, 1492.5318) ccw
  arc A275 (1168.178, 1498.5318) -> (1162.178, 1492.5318) centre (1168.178, 1492.5318) ccw
  arc A276 (1519.8447, 1430.8651) -> (1513.8447, 1436.8651) centre (1513.8447, 1430.8651) ccw
  arc A277 (1513.5113, 1313.5318) -> (1507.5113, 1307.5318) centre (1513.5113, 1307.5318) ccw
  arc A278 (1513.8447, 1313.5318) -> (1519.8447, 1319.5318) centre (1513.8447, 1319.5318) ccw
  line L311 (1551.2179, 1481.0498) -> (1787.8846, 1481.0498)
  line L312 (1787.8846, 1871.0498) -> (1551.2179, 1871.0498)
  line L313 (1792.8846, 1486.0498) -> (1792.8846, 1866.0498)
  line L314 (1546.2179, 1866.0498) -> (1546.2179, 1486.0498)
  arc A279 (1546.2179, 1486.0538) -> (1551.2187, 1481.0498) centre (1551.2179, 1486.0498) ccw
  arc A280 (1787.8806, 1481.0498) -> (1792.8846, 1486.0494) centre (1787.8846, 1486.0498) ccw
  arc A281 (1792.8846, 1866.0471) -> (1787.885, 1871.0498) centre (1787.8846, 1866.0498) ccw
  arc A282 (1551.2219, 1871.0498) -> (1546.2179, 1866.0502) centre (1551.2179, 1866.0498) ccw
  line L315 (1719.6009, 1449.2447) -> (1602.4479, 1449.2447)
  circle A283 centre (1679.5244, 1424.1256) radius 1.5
  circle A284 centre (1679.5244, 1388.8875) radius 1.5
  circle A285 centre (1642.5244, 1388.8875) radius 1.5
  circle A286 centre (1642.5244, 1406.5066) radius 1.5
  circle A287 centre (1642.5244, 1424.1256) radius 1.5
  circle A288 centre (1679.5244, 1406.5066) radius 1.5
  line L316 (1545.7813, 1325.9113) -> (1776.2676, 1325.9113)
  line L317 (1597.9758, 1446.4807) -> (1541.3091, 1333.1474)
  line L318 (1780.7397, 1333.1474) -> (1724.0731, 1446.4807)
  arc A289 (1541.3144, 1333.1578) -> (1545.7868, 1325.9114) centre (1545.7813, 1330.9113) ccw
  arc A290 (1776.2559, 1325.9114) -> (1780.7372, 1333.1524) centre (1776.2676, 1330.9113) ccw
  arc A291 (1602.4515, 1449.2447) -> (1597.9753, 1446.4798) centre (1602.4479, 1444.2447) ccw
  arc A292 (1724.0747, 1446.4775) -> (1719.5999, 1449.2447) centre (1719.6009, 1444.2447) ccw
  circle A293 centre (1248.4117, 1215.843) radius 2.5
  line L319 (1260.9117, 1228.843) -> (1235.9117, 1228.843)
  line L320 (1280.4117, 1200.843) -> (1260.9117, 1228.843)
  line L321 (1216.4117, 1200.843) -> (1280.4117, 1200.843)
  line L322 (1235.9117, 1228.843) -> (1216.4117, 1200.843)
  circle A294 centre (1250.6719, 1153.1854) radius 2.5
  line L323 (1263.1719, 1166.1854) -> (1238.1719, 1166.1854)
  line L324 (1282.6719, 1138.1854) -> (1263.1719, 1166.1854)
  line L325 (1218.6719, 1138.1854) -> (1282.6719, 1138.1854)
  line L326 (1238.1719, 1166.1854) -> (1218.6719, 1138.1854)
  line L327 (1473.2493, 921.184) -> (1283.9233, 921.184)
  line L328 (1283.9233, 921.184) -> (1271.1593, 946.7119)
  arc A295 (1280.1036, 961.184) -> (1271.1593, 946.7119) centre (1280.1036, 951.184) ccw
  line L329 (1280.1036, 961.184) -> (1447.0689, 961.184)
  arc A296 (1456.0132, 955.6562) -> (1447.0689, 961.184) centre (1447.0689, 951.184) ccw
  line L330 (1473.2493, 921.184) -> (1456.0132, 955.6562)
  circle A297 centre (1441.2493, 936.184) radius 2.5
  arc A298 (1286.2017, 950.2411) -> (1285.626, 949.5864) centre (1286.127, 949.7264) ccw
  line L331 (1290.3, 949.6464) -> (1286.2017, 950.2411)
  arc A299 (1291.5888, 946.1293) -> (1290.3, 949.6464) centre (1289.9943, 947.5397) ccw
  arc A300 (1291.5888, 946.1293) -> (1285.9645, 937.9775) centre (1295.5239, 937.3982) ccw
  arc A301 (1285.9645, 937.9775) -> (1291.5888, 929.9223) centre (1294.6348, 938.0402) ccw
  arc A302 (1291.5888, 929.9223) -> (1300.5123, 928.1077) centre (1300.7306, 952.0299) ccw
  arc A303 (1300.5123, 928.1077) -> (1301.5346, 932.9708) centre (1300.753, 930.5961) ccw
  line L332 (1301.5346, 932.9708) -> (1292.3827, 935.983)
  arc A304 (1294.0467, 941.3574) -> (1292.3827, 935.983) centre (1295.1753, 938.0633) ccw
  line L333 (1294.0467, 941.3574) -> (1297.8649, 940.215)
  arc A305 (1297.8649, 940.215) -> (1299.5798, 945.177) centre (1298.618, 942.7321) ccw
  line L334 (1299.5798, 945.177) -> (1298.0284, 945.7872)
  arc A306 (1297.8649, 948.4696) -> (1298.0284, 945.7872) centre (1298.5709, 947.1665) ccw
  line L335 (1297.8649, 948.4696) -> (1302.668, 947.4415)
  arc A307 (1306.0339, 944.0773) -> (1302.668, 947.4415) centre (1301.7512, 943.1583) ccw
  line L336 (1306.0339, 944.0773) -> (1308.0489, 934.6861)
  arc A308 (1308.0489, 934.6861) -> (1313.5524, 931.2854) centre (1312.4325, 935.6267) ccw
  arc A309 (1313.5524, 931.2854) -> (1313.5524, 937.0826) centre (1312.8046, 934.184) ccw
  line L337 (1313.5524, 937.0826) -> (1312.1216, 943.7512)
  arc A310 (1312.1216, 943.7512) -> (1301.422, 953.7544) centre (1299.5798, 941.0601) ccw
  line L338 (1301.422, 953.7544) -> (1284.6799, 956.184)
  arc A311 (1284.6799, 956.184) -> (1283.1666, 945.7565) centre (1283.9233, 950.9702) ccw
  arc A312 (1283.1666, 945.7565) -> (1285.626, 949.5864) centre (1283.5257, 948.2305) ccw
  circle A313 centre (959.2207, 1304.5117) radius 2.5
  circle A314 centre (1133.514, 1269.5117) radius 2.5
  circle A315 centre (919.2207, 1319.3755) radius 2.5
  arc A316 (1147.6161, 1274.6236) -> (1083.5982, 1319.5117) centre (1083.5982, 1251.4176) ccw
  arc A317 (1118.6892, 1266.93) -> (1147.6161, 1274.6236) centre (1133.4109, 1269.8057) ccw
  arc A318 (1118.6892, 1266.93) -> (1089.0141, 1289.5117) centre (1089.0141, 1258.7225) ccw
  line L339 (955.3696, 1289.5117) -> (1089.0141, 1289.5117)